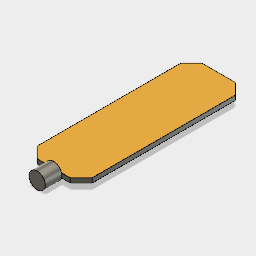
YARD Stick One v1 (Autodesk Fusion 360 design; units mm, degrees)
Autodesk Fusion 360 part; units mm, degrees
box "BoxPrimitive1" add length 60 width 20 height 1.7 placed x (0, 0, -1) y (-1, 0, 0) z (0, 1, 0) at (0, 0, 0)
chamfer "Chamfer1" distance 4 angle 45 1 edges at (-20, 0.85, 0)
chamfer "Chamfer2" distance 4 angle 45 1 edges at (0, 0.85, 0)
chamfer "Chamfer3" distance 4 angle 45 1 edges at (0, 0.85, -60)
chamfer "Chamfer4" distance 4 angle 45 1 edges at (-20, 0.85, -60)
cylinder "CylinderPrimitive1" add diameter 6 height 6 placed x (1, 0, 0) y (0, 1, 0) z (0, 0, 1) at (-10, 0.8601, 0)
